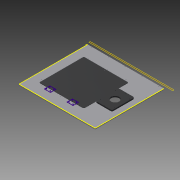
# Autodesk Inventor part: Left_side
Saved by Autodesk Inventor 2015 SP2 (Build 190223200, 223)
## iProperties
Created: 2016-11-11
Part Number: Left_side
Material: Generic
Document SubType Name: Modeling
Designer: Yann Cesbron
Density: 1 g/cm^3
Appearance: Default
Mass: 3741.54 g
Surface Area: 8542.82 cm^2
Volume: 3741.54 cm^3
Material: Perspex Black 9961 -10 mm
Author: Yann Cesbron
Autodesk Inventor part; units mm, degrees
ref_plane "YZ Plane" through (0, 0, 0) normal (1, 0, 0) x (0, 1, 0)
ref_plane "XZ Plane" through (0, 0, 0) normal (0, 1, 0) x (-1, 0, 0)
ref_plane "XY Plane" through (0, 0, 0) normal (0, 0, 1) x (1, 0, 0)
ref_plane "Work Plane1" through (11.0315, 39.8771, 0) normal (0, 0, 1) x (1, 0, 0)
sketch "Sketch1" plane through (11.0315, 39.8771, 0) normal (0, 0, 1) x (1, 0, 0)
  line L0 (-11.0315, -29.8771) -> (598.9685, -29.8771)
  line L1 (598.9685, -29.8771) -> (598.9685, -579.8771)
  line L2 (598.9685, -579.8771) -> (-11.0315, -579.8771)
  line L3 (-11.0315, -579.8771) -> (-11.0315, -29.8771)
  point P0 (-11.0315, -39.8771)
  dimension "d0" = 610
  dimension "d1" = 550
  dimension "d2" = 610
  dimension "d3" = 10
  constraints: 8 end point, 2 parallel, 1 horizontal, 1 perpendicular
  measures "d0" distance of L1.end L2.end
  measures "d1" distance of L0.end L1.end
  measures "d2" distance from line of point (-11.032, -39.877) L1
  measures "d3" distance from line of point (-11.032, -39.877) L0
extrude "Extrusion1" add sketch "Sketch1" along normal blind 10
sketch "Emission_port" plane through (11.0315, 39.8771, 10) normal (0, 0, 1) x (1, 0, 0)
  circle A0 centre (488.9685, -309.8771) radius 27.925
  line L0 (598.9685, -579.8771) -> (598.9685, -29.8771) projected
  line L1 (598.9685, -29.8771) -> (-11.0315, -29.8771) projected
  point P0 (-11.0315, -39.8771)
  dimension "d6" = 55.85
  dimension "d7" = 110
  dimension "d8" = 280
  constraints: 1 centre point
  measures "d6" diameter of A0
  measures "d7" distance from line of A0.centre L0
  measures "d8" distance from line of A0.centre L1
sketch "Cut_out_left" plane through (11.0315, 39.8771, 10) normal (0, 0, 1) x (1, 0, 0)
  line L0 (68.9685, -489.8771) -> (408.9685, -489.8771)
  line L1 (418.9685, -479.8771) -> (418.9685, -139.8771)
  line L2 (408.9685, -129.8771) -> (68.9685, -129.8771)
  line L3 (58.9685, -139.8771) -> (58.9685, -479.8771)
  line L4 (58.9685, -489.8771) -> (418.9685, -129.8771) construction
  line L5 (418.9685, -489.8771) -> (58.9685, -129.8771) construction
  line L6 (598.9685, -29.8771) -> (-11.0315, -29.8771) projected
  line L7 (598.9685, -579.8771) -> (598.9685, -29.8771) projected
  line L8 (448.9685, -384.8771) -> (528.9685, -384.8771)
  line L9 (538.9685, -374.8771) -> (538.9685, -244.8771)
  line L10 (528.9685, -234.8771) -> (448.9685, -234.8771)
  line L11 (438.9685, -244.8771) -> (438.9685, -374.8771)
  line L12 (438.9685, -384.8771) -> (538.9685, -234.8771) construction
  line L13 (538.9685, -384.8771) -> (438.9685, -234.8771) construction
  line L14 (-11.0315, -29.8771) -> (-11.0315, -579.8771) projected
  circle A0 centre (431.4685, -369.8771) radius 1.65
  circle A1 centre (431.4685, -249.8771) radius 1.65
  circle A2 centre (488.9685, -227.3771) radius 1.65
  circle A3 centre (488.9685, -392.3771) radius 1.65
  circle A4 centre (546.4685, -369.8771) radius 1.65
  circle A5 centre (546.4685, -249.8771) radius 1.65
  circle A6 centre (132.5685, -502.5771) radius 1.65
  circle A7 centre (164.3685, -502.5771) radius 1.65
  circle A8 centre (345.3685, -502.5771) radius 1.65
  circle A9 centre (313.5685, -502.5771) radius 1.65
  circle A10 centre (238.9685, -497.3771) radius 1.65
  circle A11 centre (88.9685, -497.3771) radius 1.65
  circle A12 centre (388.9685, -497.3771) radius 1.65
  circle A13 centre (426.4685, -459.8771) radius 1.65
  circle A14 centre (426.4685, -309.8771) radius 1.65
  circle A15 centre (426.4685, -159.8771) radius 1.65
  circle A16 centre (388.9685, -122.3771) radius 1.65
  circle A17 centre (238.9685, -122.3771) radius 1.65
  circle A18 centre (88.9685, -122.3771) radius 1.65
  circle A19 centre (51.4685, -459.8771) radius 1.65
  circle A20 centre (51.4685, -309.8771) radius 1.65
  circle A21 centre (51.4685, -159.8771) radius 1.65
  arc A22 (58.9685, -479.8771) -> (68.9685, -489.8771) centre (68.9685, -479.8771) ccw
  arc A23 (68.9685, -129.8771) -> (58.9685, -139.8771) centre (68.9685, -139.8771) ccw
  arc A24 (418.9685, -139.8771) -> (408.9685, -129.8771) centre (408.9685, -139.8771) ccw
  arc A25 (408.9685, -489.8771) -> (418.9685, -479.8771) centre (408.9685, -479.8771) ccw
  arc A26 (538.9685, -244.8771) -> (528.9685, -234.8771) centre (528.9685, -244.8771) ccw
  arc A27 (528.9685, -384.8771) -> (538.9685, -374.8771) centre (528.9685, -374.8771) ccw
  arc A28 (438.9685, -374.8771) -> (448.9685, -384.8771) centre (448.9685, -374.8771) ccw
  arc A29 (448.9685, -234.8771) -> (438.9685, -244.8771) centre (448.9685, -244.8771) ccw
  circle A30 centre (23.9685, -34.8771) radius 2.25
  circle A31 centre (158.9685, -34.8771) radius 2.25
  circle A32 centre (293.9685, -34.8771) radius 2.25
  circle A33 centre (428.9685, -34.8771) radius 2.25
  circle A34 centre (563.9685, -34.8771) radius 2.25
  point P0 (-11.0315, -39.8771)
  point P1 (238.9685, -309.8771)
  point P2 (488.9685, -309.8771)
  dimension "d11" = 280
  dimension "d12" = 180
  dimension "d13" = 100
  dimension "d14" = 150
  dimension "d17" = 280
  dimension "d18" = 360
  dimension "d19" = 360
  dimension "d20" = 110
  dimension "d21" = 160
  dimension "d22" = 20
  dimension "d23" = 70
  dimension "d24" = 60
  dimension "d25" = 3.3
  dimension "d26" = 3.3
  dimension "d27" = 3.3
  dimension "d28" = 3.3
  dimension "d29" = 3.3
  dimension "d30" = 3.3
  dimension "d31" = 7.5
  dimension "d32" = 7.5
  dimension "d33" = 7.5
  dimension "d34" = 7.5
  dimension "d35" = 7.5
  dimension "d36" = 7.5
  dimension "d37" = 15
  dimension "d38" = 15
  dimension "d39" = 15
  dimension "d40" = 15
  dimension "d41" = 50
  dimension "d42" = 50
  dimension "d104" = 3.3
  dimension "d105" = 3.3
  dimension "d106" = 3.3
  dimension "d107" = 3.3
  dimension "d108" = 12.7
  dimension "d109" = 12.7
  dimension "d110" = 12.7
  dimension "d111" = 12.7
  dimension "d112" = 31.8
  dimension "d113" = 31.8
  dimension "d115" = 73.6
  dimension "d116" = 73.6
  dimension "d117" = 3.3
  dimension "d118" = 3.3
  dimension "d119" = 3.3
  dimension "d120" = 3.3
  dimension "d121" = 3.3
  dimension "d122" = 3.3
  dimension "d123" = 3.3
  dimension "d124" = 3.3
  dimension "d125" = 3.3
  dimension "d126" = 3.3
  dimension "d127" = 3.3
  dimension "d128" = 3.3
  dimension "d129" = 7.5
  dimension "d130" = 7.5
  dimension "d131" = 7.5
  dimension "d132" = 7.5
  dimension "d133" = 7.5
  dimension "d134" = 7.5
  dimension "d135" = 7.5
  dimension "d136" = 7.5
  dimension "d137" = 7.5
  dimension "d138" = 7.5
  constraints: 35 centre point, 24 end point, 16 point on circle, 16 point on line, 16 tangent, 6 equal radius, 4 midpoint, 4 parallel, 2 horizontal, 2 perpendicular
  measures "d11" distance from line of L6 point (238.968, -309.877)
  measures "d12" distance between parallel lines of L7 L1
  measures "d13" distance of L13.end L12.end
  measures "d14" distance of L12.end L13.start
  measures "d17" distance from line of L6 point (488.968, -309.877)
  measures "d18" distance between parallel lines of L1 L3
  measures "d19" distance between parallel lines of L0 L2
  measures "d20" distance from line of L7 point (488.968, -309.877)
  measures "d21" distance between parallel lines of L7 L11
  measures "d22" distance between parallel lines of L1 L11
  measures "d23" distance between parallel lines of L14 L3
  measures "d24" distance between parallel lines of L7 L9
  measures "d25" diameter of A0
  measures "d26" diameter of A1
  measures "d27" diameter of A2
  measures "d28" diameter of A3
  measures "d29" diameter of A4
  measures "d30" diameter of A5
  measures "d31" distance from line of L11 A0.centre
  measures "d32" distance from line of L11 A1.centre
  measures "d33" distance from line of L10 A2.centre
  measures "d34" distance from line of L8 A3.centre
  measures "d35" distance from line of L9 A4.centre
  measures "d36" distance from line of L9 A5.centre
  measures "d37" distance from line of L8 A0.centre
  measures "d38" distance from line of L10 A1.centre
  measures "d39" distance from line of L10 A5.centre
  measures "d40" distance from line of L8 A4.centre
  measures "d41" distance from line of L9 A3.centre
  measures "d42" distance from line of L9 A2.centre
  measures "d104" diameter of A6
  measures "d105" diameter of A7
  measures "d106" diameter of A8
  measures "d107" diameter of A9
  measures "d108" distance from line of L0 A9.centre
  measures "d109" distance from line of L0 A8.centre
  measures "d110" distance from line of L0 A6.centre
  measures "d111" distance from line of L0 A7.centre
  measures "d112" distance of A9.centre A8.centre
  measures "d113" distance of A6.centre A7.centre
  measures "d115" distance from line of L1 A8.centre
  measures "d116" distance from line of L3 A6.centre
  measures "d117" diameter of A10
  measures "d118" diameter of A11
  measures "d119" diameter of A12
  measures "d120" diameter of A13
  measures "d121" diameter of A14
  measures "d122" diameter of A15
  measures "d123" diameter of A16
  measures "d124" diameter of A17
  measures "d125" diameter of A18
  measures "d126" diameter of A19
  measures "d127" diameter of A20
  measures "d128" diameter of A21
  measures "d129" distance from line of L0 A11.centre
  measures "d130" distance from line of L3 A19.centre
  measures "d131" distance from line of L3 A20.centre
  measures "d132" distance from line of L3 A21.centre
  measures "d133" distance from line of L2 A18.centre
  measures "d134" distance from line of L2 A17.centre
  measures "d135" distance from line of L0 A10.centre
  measures "d136" distance from line of L0 A12.centre
  measures "d137" distance from line of L1 A13.centre
  measures "d138" distance from line of L1 A14.centre
sketch "Flange_left" plane through (11.0315, 39.8771, 10) normal (0, 0, 1) x (1, 0, 0)
  line L0 (543.9685, -219.8771) -> (433.9685, -219.8771)
  line L1 (423.9685, -229.8771) -> (423.9685, -389.8771)
  line L2 (433.9685, -399.8771) -> (543.9685, -399.8771)
  line L3 (553.9685, -389.8771) -> (553.9685, -229.8771)
  line L4 (553.9685, -219.8771) -> (423.9685, -399.8771) construction
  line L5 (423.9685, -219.8771) -> (553.9685, -399.8771) construction
  line L6 (598.9685, -29.8771) -> (-11.0315, -29.8771) projected
  line L7 (598.9685, -579.8771) -> (598.9685, -29.8771) projected
  circle A0 centre (431.4685, -369.8771) radius 2.25
  circle A1 centre (431.4685, -249.8771) radius 2.25
  circle A2 centre (488.9685, -227.3771) radius 2.25
  circle A3 centre (488.9685, -392.3771) radius 2.25
  circle A4 centre (546.4685, -369.8771) radius 2.25
  circle A5 centre (546.4685, -249.8771) radius 2.25
  circle A6 centre (488.9685, -309.8771) radius 32.5
  arc A7 (543.9685, -399.8771) -> (553.9685, -389.8771) centre (543.9685, -389.8771) ccw
  arc A8 (423.9685, -389.8771) -> (433.9685, -399.8771) centre (433.9685, -389.8771) ccw
  arc A9 (433.9685, -219.8771) -> (423.9685, -229.8771) centre (433.9685, -229.8771) ccw
  arc A10 (553.9685, -229.8771) -> (543.9685, -219.8771) centre (543.9685, -229.8771) ccw
  point P0 (-11.0315, -39.8771)
  dimension "d43" = 130
  dimension "d44" = 180
  dimension "d45" = 280
  dimension "d46" = 110
  dimension "d47" = 4.5
  dimension "d48" = 4.5
  dimension "d49" = 4.5
  dimension "d50" = 4.5
  dimension "d51" = 4.5
  dimension "d52" = 4.5
  dimension "d53" = 7.5
  dimension "d54" = 7.5
  dimension "d55" = 7.5
  dimension "d56" = 7.5
  dimension "d57" = 7.5
  dimension "d58" = 7.5
  dimension "d59" = 30
  dimension "d60" = 30
  dimension "d61" = 65
  dimension "d62" = 65
  dimension "d63" = 30
  dimension "d64" = 30
  dimension "d65" = 65
  dimension "d159" = 10
  constraints: 12 end point, 11 centre point, 8 point on circle, 8 point on line, 8 tangent, 3 equal radius, 2 midpoint, 2 parallel, 1 coincident, 1 horizontal, 1 perpendicular
  measures "d43" distance of L5.end L4.end
  measures "d44" distance of L4.end L5.start
  measures "d45" distance from line of L6 point (488.968, -309.877)
  measures "d46" distance from line of L7 point (488.968, -309.877)
  measures "d47" diameter of A0
  measures "d48" diameter of A1
  measures "d49" diameter of A2
  measures "d50" diameter of A3
  measures "d51" diameter of A4
  measures "d52" diameter of A5
  measures "d53" distance from line of L1 A0.centre
  measures "d54" distance from line of L2 A3.centre
  measures "d55" distance from line of L1 A1.centre
  measures "d56" distance from line of L0 A2.centre
  measures "d57" distance from line of L3 A5.centre
  measures "d58" distance from line of L3 A4.centre
  measures "d59" distance from line of L2 A4.centre
  measures "d60" distance from line of L0 A5.centre
  measures "d61" distance from line of L3 A2.centre
  measures "d62" distance from line of L1 A3.centre
  measures "d63" distance from line of L2 A0.centre
  measures "d64" distance from line of L0 A1.centre
  measures "d65" diameter of A6
  measures "d159" radius of A7
sketch "Hinges_left" plane through (11.0315, 39.8771, 10) normal (0, 0, 1) x (1, 0, 0)
  line L0 (123.9685, -511.8771) -> (172.9685, -511.8771)
  line L1 (172.9685, -511.8771) -> (172.9685, -467.8771)
  line L2 (172.9685, -467.8771) -> (123.9685, -467.8771)
  line L3 (123.9685, -467.8771) -> (123.9685, -511.8771)
  line L4 (304.9685, -511.8771) -> (353.9685, -511.8771)
  line L5 (353.9685, -511.8771) -> (353.9685, -467.8771)
  line L6 (353.9685, -467.8771) -> (304.9685, -467.8771)
  line L7 (304.9685, -467.8771) -> (304.9685, -511.8771)
  line L8 (598.9685, -579.8771) -> (-11.0315, -579.8771) projected
  line L9 (598.9685, -579.8771) -> (598.9685, -29.8771) projected
  line L10 (-11.0315, -29.8771) -> (-11.0315, -579.8771) projected
  circle A0 centre (132.5685, -502.5771) radius 2.25
  circle A1 centre (164.3685, -502.5771) radius 2.25
  circle A2 centre (164.3685, -477.1771) radius 2.25
  circle A3 centre (132.5685, -477.1771) radius 2.25
  circle A4 centre (313.5685, -502.5771) radius 2.25
  circle A5 centre (345.3685, -502.5771) radius 2.25
  circle A6 centre (345.3685, -477.1771) radius 2.25
  circle A7 centre (313.5685, -477.1771) radius 2.25
  point P0 (-11.0315, -39.8771)
  dimension "d66" = 49
  dimension "d67" = 44
  dimension "d68" = 49
  dimension "d69" = 44
  dimension "d77" = 68
  dimension "d78" = 245
  dimension "d79" = 135
  dimension "d80" = 4.5
  dimension "d81" = 4.5
  dimension "d82" = 4.5
  dimension "d83" = 4.5
  dimension "d84" = 4.5
  dimension "d85" = 4.5
  dimension "d86" = 4.5
  dimension "d87" = 4.5
  dimension "d88" = 9.3
  dimension "d89" = 9.3
  dimension "d90" = 9.3
  dimension "d91" = 9.3
  dimension "d92" = 9.3
  dimension "d93" = 9.3
  dimension "d94" = 9.3
  dimension "d95" = 9.3
  dimension "d96" = 8.6
  dimension "d97" = 8.6
  dimension "d98" = 8.6
  dimension "d99" = 8.6
  dimension "d100" = 8.6
  dimension "d101" = 8.6
  dimension "d102" = 8.6
  dimension "d103" = 8.6
  constraints: 16 end point, 8 centre point, 4 parallel, 2 horizontal, 2 perpendicular, 1 point on line
  measures "d66" distance of L2.end L1.end
  measures "d67" distance of L1.end L0.end
  measures "d68" distance of L6.end L5.end
  measures "d69" distance of L5.end L4.end
  measures "d77" distance between parallel lines of L8 L0
  measures "d78" distance between parallel lines of L9 L5
  measures "d79" distance between parallel lines of L3 L10
  measures "d80" diameter of A0
  measures "d81" diameter of A1
  measures "d82" diameter of A2
  measures "d83" diameter of A3
  measures "d84" diameter of A4
  measures "d85" diameter of A5
  measures "d86" diameter of A6
  measures "d87" diameter of A7
  measures "d88" distance from line of L0 A0.centre
  measures "d89" distance from line of L0 A1.centre
  measures "d90" distance from line of L2 A2.centre
  measures "d91" distance from line of L2 A3.centre
  measures "d92" distance from line of L4 A5.centre
  measures "d93" distance from line of A4.centre L4
  measures "d94" distance from line of L6 A7.centre
  measures "d95" distance from line of L6 A6.centre
  measures "d96" distance from line of L7 A4.centre
  measures "d97" distance from line of L7 A7.centre
  measures "d98" distance from line of L5 A5.centre
  measures "d99" distance from line of L5 A6.centre
  measures "d100" distance from line of L3 A0.centre
  measures "d101" distance from line of L3 A3.centre
  measures "d102" distance from line of L1 A2.centre
  measures "d103" distance from line of L1 A1.centre
sketch "Door_left" plane through (11.0315, 39.8771, 10) normal (0, 0, 1) x (1, 0, 0)
  line L0 (68.9685, -487.8771) -> (408.9685, -487.8771)
  line L1 (416.9685, -479.8771) -> (416.9685, -139.8771)
  line L2 (408.9685, -131.8771) -> (68.9685, -131.8771)
  line L3 (60.9685, -139.8771) -> (60.9685, -479.8771)
  line L4 (60.9685, -487.8771) -> (416.9685, -131.8771) construction
  line L5 (416.9685, -487.8771) -> (60.9685, -131.8771) construction
  line L6 (598.9685, -29.8771) -> (-11.0315, -29.8771) projected
  line L7 (598.9685, -579.8771) -> (598.9685, -29.8771) projected
  arc A0 (60.9685, -479.8771) -> (68.9685, -487.8771) centre (68.9685, -479.8771) ccw
  arc A1 (408.9685, -487.8771) -> (416.9685, -479.8771) centre (408.9685, -479.8771) ccw
  arc A2 (416.9685, -139.8771) -> (408.9685, -131.8771) centre (408.9685, -139.8771) ccw
  arc A3 (68.9685, -131.8771) -> (60.9685, -139.8771) centre (68.9685, -139.8771) ccw
  circle A4 centre (132.5685, -477.1771) radius 1.65
  circle A5 centre (164.3685, -477.1771) radius 1.65
  circle A6 centre (345.3685, -477.1771) radius 1.65
  circle A7 centre (313.5685, -477.1771) radius 1.65
  point P0 (-11.0315, -39.8771)
  point P1 (238.9685, -309.8771)
  dimension "d153" = 356
  dimension "d154" = 356
  dimension "d155" = 280
  dimension "d156" = 360
  dimension "d160" = 8
  dimension "d161" = 3.3
  dimension "d162" = 3.3
  dimension "d163" = 3.3
  dimension "d164" = 3.3
  dimension "d165" = 71.6
  dimension "d166" = 10.7
  dimension "d167" = 31.8
  dimension "d168" = 10.7
  dimension "d169" = 10.7
  dimension "d170" = 10.7
  dimension "d171" = 31.8
  dimension "d172" = 71.6
  constraints: 12 end point, 8 centre point, 8 point on circle, 8 point on line, 8 tangent, 3 equal radius, 2 midpoint, 2 parallel, 1 horizontal, 1 perpendicular
  measures "d153" distance of L5.end L4.end
  measures "d154" distance of L4.end L5.start
  measures "d155" distance from line of L6 point (238.968, -309.877)
  measures "d156" distance from line of L7 point (238.968, -309.877)
  measures "d160" radius of A0
  measures "d161" diameter of A4
  measures "d162" diameter of A5
  measures "d163" diameter of A6
  measures "d164" diameter of A7
  measures "d165" distance from line of L1 A6.centre
  measures "d166" distance from line of L0 A6.centre
  measures "d167" distance of A7.centre A6.centre
  measures "d168" distance from line of L0 A7.centre
  measures "d169" distance from line of L0 A5.centre
  measures "d170" distance from line of L0 A4.centre
  measures "d171" distance of A5.centre A4.centre
  measures "d172" distance from line of L3 A4.centre
sketch "Panel_left_holes_left" plane through (0, -540, 0) normal (0, -1, 0) x (1, 0, 0)
  circle A0 centre (575, 5) radius 1.65
  circle A1 centre (440, 5) radius 1.65
  circle A2 centre (305, 5) radius 1.65
  circle A3 centre (170, 5) radius 1.65
  circle A4 centre (35, 5) radius 1.65
  line L0 (0, 10) -> (610, 10) projected
  line L1 (0, 0) -> (0, 10) projected
  line L2 (610, 0) -> (610, 10) projected
  dimension "d188" = 3.3
  dimension "d189" = 3.3
  dimension "d190" = 3.3
  dimension "d191" = 3.3
  dimension "d192" = 3.3
  dimension "d193" = 5
  dimension "d194" = 35
  dimension "d195" = 5
  dimension "d196" = 5
  dimension "d197" = 5
  dimension "d198" = 135
  dimension "d199" = 5
  dimension "d200" = 35
  dimension "d201" = 135
  dimension "d202" = 135
  constraints: 5 centre point
  measures "d188" diameter of A0
  measures "d189" diameter of A1
  measures "d190" diameter of A2
  measures "d191" diameter of A3
  measures "d192" diameter of A4
  measures "d193" distance from line of L0 A4.centre
  measures "d194" distance from line of L1 A4.centre
  measures "d195" distance from line of L0 A3.centre
  measures "d196" distance from line of L0 A2.centre
  measures "d197" distance from line of L0 A1.centre
  measures "d198" distance of A3.centre A4.centre
  measures "d199" distance from line of L0 A0.centre
  measures "d200" distance from line of L2 A0.centre
  measures "d201" distance of A1.centre A0.centre
  measures "d202" distance of A2.centre A1.centre
sketch "Panel_top_holes_left" plane through (0, -540, 0) normal (-1, 0, 0) x (0, 0, 1)
  circle A0 centre (5, 515) radius 1.65
  circle A1 centre (5, 355) radius 1.65
  circle A2 centre (5, 195) radius 1.65
  circle A3 centre (5, 35) radius 1.65
  line L0 (10, 550) -> (10, 0) projected
  line L1 (0, 0) -> (10, 0) projected
  line L2 (0, 550) -> (10, 550) projected
  point P0 (0, 540)
  dimension "d203" = 3.3
  dimension "d204" = 3.3
  dimension "d205" = 3.3
  dimension "d206" = 3.3
  dimension "d207" = 5
  dimension "d208" = 35
  dimension "d209" = 5
  dimension "d210" = 160
  dimension "d211" = 5
  dimension "d212" = 35
  dimension "d213" = 5
  dimension "d214" = 160
  dimension "d215" = 160
  constraints: 4 centre point
  measures "d203" diameter of A0
  measures "d204" diameter of A1
  measures "d205" diameter of A2
  measures "d206" diameter of A3
  measures "d207" distance from line of L0 A3.centre
  measures "d208" distance from line of L1 A3.centre
  measures "d209" distance from line of L0 A2.centre
  measures "d210" distance of A2.centre A3.centre
  measures "d211" distance from line of L0 A0.centre
  measures "d212" distance from line of A0.centre L2
  measures "d213" distance from line of L0 A1.centre
  measures "d214" distance of A0.centre A1.centre
  measures "d215" distance of A2.centre A1.centre
extrude "Extrusion2" cut sketch "Cut_out_left" against normal blind 10
extrude "Extrusion3" add sketch "Door_left" against normal blind 10 separate body
extrude "Extrusion4" add sketch "Flange_left" along normal blind 10 separate body
extrude "Extrusion5" cut sketch "Panel_left_holes_left" against normal blind 15 bodies 1
extrude "Extrusion6" cut sketch "Panel_top_holes_left" against normal blind 15 bodies 1
sketch "Door_hole_left" plane through (11.0315, 39.8771, 0) normal (0, 0, -1) x (-1, 0, 0)
  line L0 (-416.9685, -139.8771) -> (-416.9685, -479.8771) projected
  line L1 (-68.9685, -131.8771) -> (-408.9685, -131.8771) projected
  point P0 (11.0315, -39.8771)
  point P1 (-238.9685, -144.8771)
  dimension "d235" = 178
  dimension "d236" = 13
  measures "d235" distance from line of L0 point (-238.968, -144.877)
  measures "d236" distance from line of L1 point (-238.968, -144.877)
hole "CSK_Door_hole_left" at (250, -105, 0) direction (0, 0, 1) diameter 7 end through all countersink diameter 12.6 countersink angle 90 bodies 2 clearance for "Countersunk Flat Head Screw DIN EN ISO 2009" size "M6" standard "DIN"
sketch "Door_flanges_left" plane through (11.0315, 39.8771, 0) normal (0, 0, -1) x (-1, 0, 0)
  line L0 (-433.9685, -139.8771) -> (-433.9685, -114.8771)
  line L1 (-433.9685, -114.8771) -> (-43.9685, -114.8771)
  line L2 (-43.9685, -114.8771) -> (-43.9685, -139.8771)
  line L3 (-408.9685, -129.8771) -> (-68.9685, -129.8771) projected
  line L4 (-58.9685, -139.8771) -> (-58.9685, -479.8771) projected
  line L5 (-418.9685, -479.8771) -> (-418.9685, -139.8771) projected
  line L6 (-43.9685, -504.8771) -> (-433.9685, -504.8771)
  line L7 (-433.9685, -504.8771) -> (-433.9685, -479.8771)
  line L8 (-433.9685, -479.8771) -> (-43.9685, -479.8771)
  line L9 (-43.9685, -479.8771) -> (-43.9685, -504.8771)
  line L10 (-68.9685, -489.8771) -> (-408.9685, -489.8771) projected
  line L11 (-433.9685, -140.8771) -> (-408.9685, -140.8771)
  line L12 (-408.9685, -140.8771) -> (-408.9685, -478.8771)
  line L13 (-408.9685, -478.8771) -> (-433.9685, -478.8771)
  line L14 (-433.9685, -478.8771) -> (-433.9685, -140.8771)
  line L15 (-43.9685, -140.8771) -> (-68.9685, -140.8771)
  line L16 (-68.9685, -140.8771) -> (-68.9685, -478.8771)
  line L17 (-68.9685, -478.8771) -> (-43.9685, -478.8771)
  line L18 (-43.9685, -478.8771) -> (-43.9685, -140.8771)
  circle A0 centre (-51.4685, -459.8771) radius 2.25
  circle A1 centre (-51.4685, -309.8771) radius 2.25
  circle A2 centre (-51.4685, -159.8771) radius 2.25
  circle A3 centre (-88.9685, -497.3771) radius 2.25
  circle A4 centre (-88.9685, -122.3771) radius 2.25
  circle A5 centre (-238.9685, -122.3771) radius 2.25
  circle A6 centre (-388.9685, -122.3771) radius 2.25
  circle A7 centre (-426.4685, -159.8771) radius 2.25
  circle A8 centre (-426.4685, -309.8771) radius 2.25
  circle A9 centre (-426.4685, -459.8771) radius 2.25
  circle A10 centre (-388.9685, -497.3771) radius 2.25
  circle A11 centre (-238.9685, -497.3771) radius 2.25
  line L19 (-228.9685, -131.8771) -> (-248.9685, -131.8771)
  line L20 (-248.9685, -131.8771) -> (-248.9685, -139.8771)
  line L21 (-228.9685, -139.8771) -> (-228.9685, -131.8771)
  line L22 (-43.9685, -139.8771) -> (-228.9685, -139.8771)
  line L23 (-248.9685, -139.8771) -> (-433.9685, -139.8771)
  circle A12 centre (-221.4685, -132.3771) radius 1.65
  circle A13 centre (-256.4685, -132.3771) radius 1.65
  point P0 (11.0315, -39.8771)
  dimension "d244" = 390
  dimension "d245" = 25
  dimension "d247" = 15
  dimension "d249" = 390
  dimension "d250" = 25
  dimension "d251" = 15
  dimension "d252" = 10
  dimension "d253" = 25
  dimension "d256" = 10
  dimension "d259" = 338
  dimension "d260" = 25
  dimension "d261" = 338
  dimension "d263" = 15
  dimension "d264" = 4.5
  dimension "d265" = 4.5
  dimension "d266" = 4.5
  dimension "d267" = 4.5
  dimension "d268" = 4.5
  dimension "d269" = 4.5
  dimension "d270" = 4.5
  dimension "d271" = 4.5
  dimension "d272" = 4.5
  dimension "d273" = 4.5
  dimension "d274" = 4.5
  dimension "d275" = 4.5
  dimension "d276" = 7.5
  dimension "d277" = 45
  dimension "d278" = 7.5
  dimension "d280" = 7.5
  dimension "d281" = 7.5
  dimension "d282" = 7.5
  dimension "d283" = 19
  dimension "d284" = 45
  dimension "d285" = 19
  dimension "d286" = 150
  dimension "d287" = 7.5
  dimension "d288" = 7.5
  dimension "d289" = 7.5
  dimension "d290" = 19
  dimension "d291" = 150
  dimension "d292" = 7.5
  dimension "d293" = 45
  dimension "d294" = 7.5
  dimension "d295" = 150
  dimension "d296" = 19
  dimension "d297" = 7.5
  dimension "d298" = 7.5
  dimension "d300" = 45
  dimension "d301" = 150
  dimension "d388" = 25
  dimension "d389" = 1
  dimension "d390" = 1
  dimension "d391" = 20
  dimension "d392" = 185
  dimension "d393" = 8
  dimension "d394" = 15
  dimension "d395" = 3.3
  dimension "d396" = 3.3
  dimension "d397" = 7.5
  dimension "d398" = 7.5
  dimension "d399" = 7.5
  dimension "d400" = 7.5
  constraints: 40 end point, 14 centre point, 10 parallel, 6 horizontal, 6 perpendicular
  measures "d244" distance of L0.end L1.end
  measures "d245" distance of L0.start L0.end
  measures "d247" distance between parallel lines of L4 L2
  measures "d249" distance of L7.end L8.end
  measures "d250" distance of L6.end L7.end
  measures "d251" distance between parallel lines of L4 L9
  measures "d252" distance between parallel lines of L10 L8
  measures "d253" distance of L12.end L13.end
  measures "d256" distance between parallel lines of L5 L12
  measures "d259" distance between parallel lines of L11 L13
  measures "d260" distance of L17.end L16.end
  measures "d261" distance of L16.end L15.end
  measures "d263" distance between parallel lines of L4 L18
  measures "d264" diameter of A0
  measures "d265" diameter of A1
  measures "d266" diameter of A2
  measures "d267" diameter of A3
  measures "d268" diameter of A4
  measures "d269" diameter of A5
  measures "d270" diameter of A6
  measures "d271" diameter of A7
  measures "d272" diameter of A8
  measures "d273" diameter of A9
  measures "d274" diameter of A10
  measures "d275" diameter of A11
  measures "d276" distance from line of L6 A3.centre
  measures "d277" distance from line of L9 A3.centre
  measures "d278" distance from line of L18 A0.centre
  measures "d280" distance from line of L18 A1.centre
  measures "d281" distance from line of L18 A2.centre
  measures "d282" distance from line of L1 A4.centre
  measures "d283" distance from line of L15 A2.centre
  measures "d284" distance from line of L2 A4.centre
  measures "d285" distance from line of L17 A0.centre
  measures "d286" distance of A1.centre A2.centre
  measures "d287" distance from line of L14 A7.centre
  measures "d288" distance from line of L14 A8.centre
  measures "d289" distance from line of L14 A9.centre
  measures "d290" distance from line of L11 A7.centre
  measures "d291" distance of A8.centre A7.centre
  measures "d292" distance from line of L1 A6.centre
  measures "d293" distance from line of L0 A6.centre
  measures "d294" distance from line of L1 A5.centre
  measures "d295" distance of A5.centre A6.centre
  measures "d296" distance from line of L13 A9.centre
  measures "d297" distance from line of L6 A10.centre
  measures "d298" distance from line of L6 A11.centre
  measures "d300" distance from line of L7 A10.centre
  measures "d301" distance of A3.centre A11.centre
  measures "d388" distance between parallel lines of L22 L1
  measures "d389" distance between parallel lines of L15 L22
  measures "d390" distance between parallel lines of L8 L13
  measures "d391" distance between parallel lines of L20 L21
  measures "d392" distance from line of L19.end L0
  measures "d393" distance between parallel lines of L22 L19
  measures "d394" distance between parallel lines of L1 L3
  measures "d395" diameter of A12
  measures "d396" diameter of A13
  measures "d397" distance from line of L23 A13.centre
  measures "d398" distance from line of L22 A12.centre
  measures "d399" distance from line of L21 A12.centre
  measures "d400" distance from line of L20 A13.centre
extrude "Door_flanges_left_1" add sketch "Door_flanges_left" along normal blind 10 separate body contours L8 L9 L6 L7
extrude "Door_flanges_left_2" add sketch "Door_flanges_left" along normal blind 10 separate body contours L11 L12 L13 L5 | L5 L13 L14 L11
extrude "Door_flanges_left_3" add sketch "Door_flanges_left" along normal blind 10 separate body contours L15 L18 L17 L4 | L4 L17 L16 L15
extrude "Door_flanges_left_4" add sketch "Door_flanges_left" along normal blind 10 separate body contours L0 L1 L2 L22 L21 L19 L20 L23
sketch "Magnet_flange_left" plane through (11.0315, 39.8771, -10) normal (0, 0, -1) x (-1, 0, 0)
  circle A0 centre (-238.9685, -144.8771) radius 1.65
  arc A1 (-244.9685, -124.8771) -> (-232.9685, -124.8771) centre (-238.9685, -124.8771) ccw
  line L0 (-248.9685, -154.8771) -> (-228.9685, -154.8771)
  line L1 (-248.9685, -154.8771) -> (-248.9685, -139.8771)
  circle A2 centre (-256.4685, -132.3771) radius 2.25
  line L2 (-248.9685, -139.8771) -> (-263.9685, -139.8771)
  line L3 (-263.9685, -124.8771) -> (-263.9685, -139.8771)
  line L4 (-244.9685, -124.8771) -> (-263.9685, -124.8771)
  line L5 (-228.9685, -154.8771) -> (-228.9685, -139.8771)
  circle A3 centre (-221.4685, -132.3771) radius 2.25
  line L6 (-213.9685, -124.8771) -> (-232.9685, -124.8771)
  line L7 (-213.9685, -139.8771) -> (-213.9685, -124.8771)
  line L8 (-228.9685, -139.8771) -> (-213.9685, -139.8771)
  point P0 (11.0315, -39.8771)
  dimension "d409" = 50
  dimension "d410" = 15
  dimension "d411" = 15
  dimension "d412" = 15
  dimension "d413" = 4.5
  dimension "d414" = 4.5
  dimension "d415" = 7.5
  dimension "d416" = 7.5
  dimension "d417" = 12
  dimension "d418" = 15
  dimension "d419" = 15
  dimension "d420" = 7.5
  dimension "d421" = 7.5
  dimension "d422" = 19
  dimension "d423" = 3.3
  dimension "d424" = 10
  dimension "d425" = 10
  constraints: 18 end point, 4 centre point, 3 parallel, 3 perpendicular, 2 line through centre, 2 point on circle, 1 coincident, 1 horizontal
  measures "d409" distance between parallel lines of L7 L3
  measures "d410" distance between parallel lines of L3 L1
  measures "d411" distance between parallel lines of L7 L5
  measures "d412" distance between parallel lines of L0 L2
  measures "d413" diameter of A2
  measures "d414" diameter of A3
  measures "d415" distance from line of L3 A2.centre
  measures "d416" distance from line of L7 A3.centre
  measures "d417" diameter of A1
  measures "d418" distance between parallel lines of L4 L2
  measures "d419" distance between parallel lines of L6 L8
  measures "d420" distance from line of L2 A2.centre
  measures "d421" distance from line of L8 A3.centre
  measures "d422" distance of L4.start L3.start
  measures "d423" diameter of A0
  measures "d424" distance from line of L1 A0.centre
  measures "d425" distance from line of L0 A0.centre
extrude "Magnet_flange_left_1" add sketch "Magnet_flange_left" along normal blind 10 separate body
sketch "Bracket_holes_left" plane through (11.0315, 39.8771, 10) normal (0, 0, 1) x (1, 0, 0)
  line L0 (598.9685, -579.8771) -> (598.9685, -29.8771) projected
  line L1 (-11.0315, -579.8771) -> (598.9685, -579.8771) projected
  line L2 (598.9685, -29.8771) -> (-11.0315, -29.8771) projected
  point P0 (-11.0315, -39.8771)
  point P1 (591.4685, -159.8771)
  point P2 (591.4685, -459.8771)
  dimension "d438" = 7.5
  dimension "d439" = 7.5
  dimension "d440" = 120
  dimension "d441" = 130
  measures "d438" distance from line of L0 point (591.468, -159.877)
  measures "d439" distance from line of L0 point (591.468, -459.877)
  measures "d440" distance from line of L1 point (591.468, -459.877)
  measures "d441" distance from line of L2 point (591.468, -159.877)
hole "Bracket_holes_left_1" at (602.5, -120, 10) at (602.5, -420, 10) direction (0, 0, -1) diameter 3.3 end through all bodies 1
